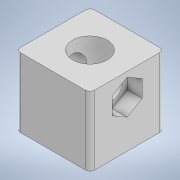
# Autodesk Inventor part: Spoolsupport
Saved by Autodesk Inventor 2020.2 (Build 242310000, 310)
## iProperties
Created: 2020-07-31
Part Number: Spoolsupport
Material: Generic
Document SubType Name: Modeling
Designer: JK
Density: 1 g/cm^3
Appearance: Default
Author: JK
Autodesk Inventor part; units mm, degrees
ref_plane "YZ Plane" through (0, 0, 0) normal (1, 0, 0) x (0, 1, 0)
ref_plane "XZ Plane" through (0, 0, 0) normal (0, 1, 0) x (-1, 0, 0)
ref_plane "XY Plane" through (0, 0, 0) normal (0, 0, 1) x (1, 0, 0)
sketch "Sketch1" plane through (0, 0, 0) normal (0, 1, 0) x (-1, 0, 0)
  line L0 (-15, 15) -> (15, 15)
  line L1 (15, 15) -> (15, -15)
  line L2 (15, -15) -> (-15, -15)
  line L3 (-15, -15) -> (-15, 15)
  line L4 (-15, 15) -> (15, -15) construction
  line L5 (15, 15) -> (-15, -15) construction
  point P0 (0, 0)
  dimension "d0" = 30
  dimension "d1" = 30
  constraints: 12 end point, 2 midpoint, 2 parallel, 1 horizontal, 1 perpendicular
  measures "d0" distance of L0.end L1.end
  measures "d1" distance of L1.end L2.end
extrude "Extrusion1" add sketch "Sketch1" along normal blind 11
sketch "Sketch2" plane through (0, 11, 0) normal (0, 1, 0) x (1, 0, 0)
  circle A0 centre (0, 0) radius 7
  dimension "d4" = 14
  constraints: 1 centre point, 1 coincident
  measures "d4" diameter of A0
extrude "Extrusion2" cut sketch "Sketch2" against normal blind 9
sketch "Sketch3" plane through (0, 11, 0) normal (0, 1, 0) x (1, 0, 0)
  circle A0 centre (0, 0) radius 7 projected
  line L0 (-15, -15) -> (15, -15) projected
  line L1 (15, -15) -> (15, 15) projected
  line L2 (15, 15) -> (-15, 15) projected
  line L3 (-15, 15) -> (-15, -15) projected
extrude "Extrusion3" add sketch "Sketch3" along normal blind 17
sketch "Sketch4" plane through (15, 0, 15) normal (1, 0, 0) x (0, 0, -1)
  circle A0 centre (15, 19) radius 4
  line L0 (0, 28) -> (30, 28) projected
  line L1 (15, 26) -> (21.0622, 22.5)
  line L2 (21.0622, 22.5) -> (21.0622, 15.5)
  line L3 (21.0622, 15.5) -> (15, 12)
  line L4 (15, 12) -> (8.9378, 15.5)
  line L5 (8.9378, 15.5) -> (8.9378, 22.5)
  line L6 (8.9378, 22.5) -> (15, 26)
  circle A1 centre (15, 19) radius 7
  point P0 (15, 0)
  dimension "d11" = 14
  dimension "d9" = 8
  dimension "d10" = 9
  constraints: 12 end point, 2 coincident, 1 centre point, 1 vertical alignment, 15 other
  measures "d9" diameter of A0
  measures "d10" distance from line of L0 A0.centre
extrude "Extrusion4" cut sketch "Sketch4" against normal blind 6 contours A0 | L1 L2 L3 L4 L5 L6
sketch "Sketch5" plane through (9, 0, 15) normal (1, 0, 0) x (0, 0, -1)
  circle A0 centre (15, 19) radius 4.25
  line L0 (0, 28) -> (30, 28) projected
  point P0 (15, 0)
  dimension "d14" = 8.5
  dimension "d20" = 9
  constraints: 1 centre point
  measures "d14" diameter of A0
  measures "d20" distance from line of L0 A0.centre
extrude "Extrusion5" cut sketch "Sketch5" against normal through all
sketch "Sketch6" plane through (0, 2, 0) normal (0, 1, 0) x (1, 0, 0)
  circle A0 centre (0, 0) radius 4.15
  dimension "d17" = 8.3
  constraints: 1 centre point, 1 coincident
  measures "d17" diameter of A0
extrude "Extrusion6" cut sketch "Sketch6" against normal through all
fillet "Fillet1" radius 2 4 edges at (15, 14, -15) (-15, 14, -15) (-15, 14, 15) (15, 14, 15)
body "Solid1"
